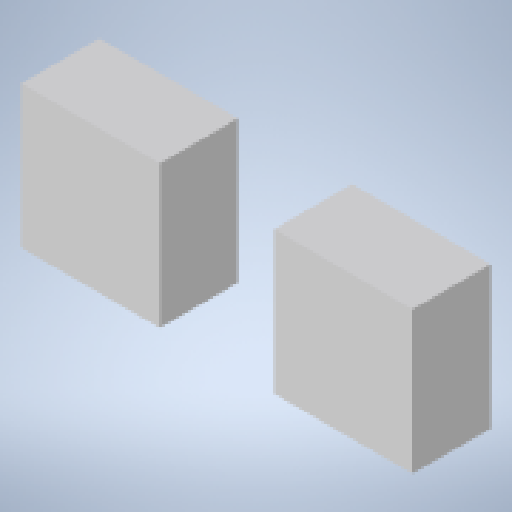
# Autodesk Inventor part: spacer1
Saved by Autodesk Inventor 2025 (Build 290162000, 162)
## iProperties
Created: 2025-05-22
Part Number: spacer1
Material: Generic
Document SubType Name: Modeling
Designer: warke
Density: 1 g/cm^3
Appearance: Default
Author: warke
Autodesk Inventor part; units mm, degrees
ref_plane "YZ Plane" through (0, 0, 0) normal (1, 0, 0) x (0, 1, 0)
ref_plane "XZ Plane" through (0, 0, 0) normal (0, 1, 0) x (-1, 0, 0)
sketch "Sketch1" plane through (0, 0, 0) normal (0, 0, 1) x (1, 0, 0)
  point P0 (0, 0)
sketch "Sketch2" plane through (0, 0, 0) normal (0, 0, 1) x (1, 0, 0)
  line L0 (-5.5, 2) -> (5.5, 2) projected
  line L1 (-5.5, -2) -> (-5.5, 2) projected
  line L2 (5.5, -2) -> (-5.5, -2) projected
  line L3 (5.5, 2) -> (5.5, -2) projected
  line L4 (-1.6, 2) -> (-1.6, -2) projected
  line L5 (1.6, -2) -> (1.6, 2) projected
  point P0 (0, 0)
ref_plane "Work Plane1" through (-5.4608, -2, 2.2) normal (0, 0, -1) x (0, 1, 0)
extrude "Extrusion1" add sketch "Sketch2" along normal up to surface (2.2 mm away) contours L0 L4 L2 L1 | L0 L3 L2 L5
body "Solid1"
